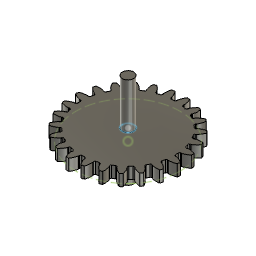
test (Autodesk Fusion 360 design; units mm, degrees)
description: Spur Gear; Module: 0.700000; Num Teeth: 26; Pressure Angle: 20.000000; Backlash: 0.00 mm
Autodesk Fusion 360 part; units mm, degrees
sketch "Sketch1" plane through (0, 0, 0) normal (0, 0, 1) x (1, 0, 0)
  circle A0 centre (0, 0) radius 8.2092
  circle A1 centre (0, 0) radius 1
extrude "Extrude1" add sketch "Sketch1" along normal blind 2 makes body 1
sketch "Sketch2" plane through (0, 0, 0) normal (0, 0, 1) x (1, 0, 0)
  spline S0 degree 5 poles (8.527, -0.6435) (8.5306, -0.6437) (8.5378, -0.6442) (8.5487, -0.6446) (8.5632, -0.6446) (8.5813, -0.644) (8.5995, -0.6429) (8.6176, -0.6415) (8.6358, -0.6399) (8.654, -0.6382) (8.6723, -0.6364) (8.6905, -0.6344) (8.7087, -0.6322) (8.7269, -0.6298) (8.7452, -0.6271) (8.7634, -0.6242) (8.7816, -0.6211) (8.7999, -0.6179) (8.8181, -0.6145) (8.8364, -0.6109) (8.8546, -0.6073) (8.8729, -0.6035) (8.8911, -0.5995) (8.9094, -0.5954) (8.9276, -0.5912) (8.9459, -0.5868) (8.9641, -0.5822) (8.9824, -0.5776) (9.0006, -0.5728) (9.0189, -0.5679) (9.0371, -0.5628) (9.0553, -0.5577) (9.0736, -0.5524) (9.0918, -0.547) (9.11, -0.5414) (9.1282, -0.5358) (9.1464, -0.53) (9.1647, -0.5242) (9.1829, -0.5182) (9.2011, -0.5121) (9.2192, -0.5059) (9.2374, -0.4995) (9.2556, -0.4931) (9.2738, -0.4866) (9.292, -0.4799) (9.3101, -0.4731) (9.3283, -0.4663) (9.3464, -0.4593) (9.3645, -0.4523) (9.3827, -0.4451) (9.4008, -0.4378) (9.4189, -0.4304) (9.437, -0.423) (9.4551, -0.4154) (9.4732, -0.4077) (9.4912, -0.3999) (9.5093, -0.3921) (9.5273, -0.3841) (9.5454, -0.376) (9.5634, -0.3679) (9.5814, -0.3596) (9.5994, -0.3513) (9.6174, -0.3428) (9.6354, -0.3343) (9.6534, -0.3257) (9.6714, -0.3169) (9.6893, -0.3081) (9.7072, -0.2992) (9.7252, -0.2902) (9.7431, -0.2811) (9.761, -0.272) (9.7753, -0.2645) (9.786, -0.2589) (9.7932, -0.2552) (9.7967, -0.2533) knots 0 0 0 0 0 0 0.01428571 0.02857143 0.04285714 0.05714286 0.07142857 0.08571429 0.1 0.11428571 0.12857143 0.14285714 0.15714286 0.17142857 0.18571429 0.2 0.21428571 0.22857143 0.24285714 0.25714286 0.27142857 0.28571429 0.3 0.31428571 0.32857143 0.34285714 0.35714286 0.37142857 0.38571429 0.4 0.41428571 0.42857143 0.44285714 0.45714286 0.47142857 0.48571429 0.5 0.51428571 0.52857143 0.54285714 0.55714286 0.57142857 0.58571429 0.6 0.61428571 0.62857143 0.64285714 0.65714286 0.67142857 0.68571429 0.7 0.71428571 0.72857143 0.74285714 0.75714286 0.77142857 0.78571429 0.8 0.81428571 0.82857143 0.84285714 0.85714286 0.87142857 0.88571429 0.9 0.91428571 0.92857143 0.94285714 0.95714286 0.97142857 0.98571429 1 1 1 1 1 1
  spline S1 degree 5 poles (8.527, 0.6435) (8.5306, 0.6437) (8.5378, 0.6442) (8.5487, 0.6446) (8.5632, 0.6446) (8.5813, 0.644) (8.5995, 0.6429) (8.6176, 0.6415) (8.6358, 0.6399) (8.654, 0.6382) (8.6723, 0.6364) (8.6905, 0.6344) (8.7087, 0.6322) (8.7269, 0.6298) (8.7452, 0.6271) (8.7634, 0.6242) (8.7816, 0.6211) (8.7999, 0.6179) (8.8181, 0.6145) (8.8364, 0.6109) (8.8546, 0.6073) (8.8729, 0.6035) (8.8911, 0.5995) (8.9094, 0.5954) (8.9276, 0.5912) (8.9459, 0.5868) (8.9641, 0.5822) (8.9824, 0.5776) (9.0006, 0.5728) (9.0189, 0.5679) (9.0371, 0.5628) (9.0553, 0.5577) (9.0736, 0.5524) (9.0918, 0.547) (9.11, 0.5414) (9.1282, 0.5358) (9.1464, 0.53) (9.1647, 0.5242) (9.1829, 0.5182) (9.2011, 0.5121) (9.2192, 0.5059) (9.2374, 0.4995) (9.2556, 0.4931) (9.2738, 0.4866) (9.292, 0.4799) (9.3101, 0.4731) (9.3283, 0.4663) (9.3464, 0.4593) (9.3645, 0.4523) (9.3827, 0.4451) (9.4008, 0.4378) (9.4189, 0.4304) (9.437, 0.423) (9.4551, 0.4154) (9.4732, 0.4077) (9.4912, 0.3999) (9.5093, 0.3921) (9.5273, 0.3841) (9.5454, 0.376) (9.5634, 0.3679) (9.5814, 0.3596) (9.5994, 0.3513) (9.6174, 0.3428) (9.6354, 0.3343) (9.6534, 0.3257) (9.6714, 0.3169) (9.6893, 0.3081) (9.7072, 0.2992) (9.7252, 0.2902) (9.7431, 0.2811) (9.761, 0.272) (9.7753, 0.2645) (9.786, 0.2589) (9.7932, 0.2552) (9.7967, 0.2533) knots 0 0 0 0 0 0 0.01428571 0.02857143 0.04285714 0.05714286 0.07142857 0.08571429 0.1 0.11428571 0.12857143 0.14285714 0.15714286 0.17142857 0.18571429 0.2 0.21428571 0.22857143 0.24285714 0.25714286 0.27142857 0.28571429 0.3 0.31428571 0.32857143 0.34285714 0.35714286 0.37142857 0.38571429 0.4 0.41428571 0.42857143 0.44285714 0.45714286 0.47142857 0.48571429 0.5 0.51428571 0.52857143 0.54285714 0.55714286 0.57142857 0.58571429 0.6 0.61428571 0.62857143 0.64285714 0.65714286 0.67142857 0.68571429 0.7 0.71428571 0.72857143 0.74285714 0.75714286 0.77142857 0.78571429 0.8 0.81428571 0.82857143 0.84285714 0.85714286 0.87142857 0.88571429 0.9 0.91428571 0.92857143 0.94285714 0.95714286 0.97142857 0.98571429 1 1 1 1 1 1
  arc A0 (9.7967, -0.2533) -> (9.7967, 0.2533) centre (0, 0) ccw
  line L0 (8.176, -0.6177) -> (8.527, -0.6435)
  line L1 (8.176, 0.6177) -> (8.527, 0.6435)
  line L2 (8.176, -0.6177) -> (8.176, 0.6177)
  point P0 (8.6166, -0.6416)
  point P1 (8.7067, -0.6324)
  point P2 (8.7971, -0.6183)
  point P3 (8.8878, -0.6002)
  point P4 (8.9786, -0.5785)
  point P5 (9.0695, -0.5535)
  point P6 (9.1605, -0.5255)
  point P7 (9.2516, -0.4945)
  point P8 (9.3426, -0.4607)
  point P9 (9.4337, -0.4243)
  point P10 (9.5246, -0.3853)
  point P11 (9.6155, -0.3437)
  point P12 (9.7062, -0.2997)
  point P13 (8.6166, 0.6416)
  point P14 (8.7067, 0.6324)
  point P15 (8.7971, 0.6183)
  point P16 (8.8878, 0.6002)
  point P17 (8.9786, 0.5785)
  point P18 (9.0695, 0.5535)
  point P19 (9.1605, 0.5255)
  point P20 (9.2516, 0.4945)
  point P21 (9.3426, 0.4607)
  point P22 (9.4337, 0.4243)
  point P23 (9.5246, 0.3853)
  point P24 (9.6155, 0.3437)
  point P25 (9.7062, 0.2997)
extrude "Extrude2" add sketch "Sketch2" along normal blind 2 bodies 1
fillet "Fillet1" radius 0.2 2 edges at (8.1859, -0.6185, 1) (8.1859, 0.6185, 1) on bodies 1
pattern_circular "C-Pattern1" count 24 over 360 about axis through (0, 0, 0) along (0, 0, 1) of "Extrude2", "Fillet1"
sketch "Sketch3" plane through (0, 0, 0) normal (0, 0, 1) x (1, 0, 0)
  circle A0 centre (0, 0) radius 9.1 construction
sketch "sketch 667" plane through (0, 44, 2) normal (0, 0, 1) x (-1, 0, 0)
  circle A0 centre (0, 44) radius 1
extrude "Extrude3" add sketch "sketch 667" along normal mid plane 16 separate body makes body 2
move_body "Move1" bodies 1 to x (0.984808, 0.173648, 0) y (-0.173648, 0.984808, 0) z (0, 0, 1) at (0, 0, 0)
